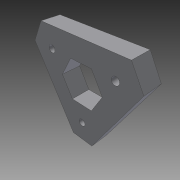
# Autodesk Inventor part: spool_hex_holder
Saved by Autodesk Inventor 2014 (Build 180170000, 170)
## iProperties
Created: 2014-04-15
Part Number: spool_hex_holder
Material: Plywood, Finish
Document SubType Name: Modeling
Designer: buben
Density: 0.552 g/cm^3
Appearance: Plywood - New
Author: buben
Autodesk Inventor part; units mm, degrees
ref_plane "YZ Plane" through (0, 0, 0) normal (1, 0, 0) x (0, 1, 0)
ref_plane "XZ Plane" through (0, 0, 0) normal (0, 1, 0) x (-1, 0, 0)
ref_plane "XY Plane" through (0, 0, 0) normal (0, 0, 1) x (1, 0, 0)
sketch "Sketch1" plane through (0, 0, 0) normal (0, 1, 0) x (-1, 0, 0)
  line L0 (-3.7528, 6.5) -> (3.7528, 6.5)
  line L1 (3.7528, 6.5) -> (7.5056, 0)
  line L2 (7.5056, 0) -> (3.7528, -6.5)
  line L3 (3.7528, -6.5) -> (-3.7528, -6.5)
  line L4 (-3.7528, -6.5) -> (-7.5056, 0)
  line L5 (-7.5056, 0) -> (-3.7528, 6.5)
  line L6 (-15.0363, 13.3) -> (15.0363, 13.3)
  line L7 (19.0363, 6.3718) -> (4, -19.6718)
  line L8 (-4, -19.6718) -> (-19.0363, 6.3718)
  line L9 (19.0363, 6.3718) -> (15.0363, 13.3)
  line L10 (-15.0363, 13.3) -> (-19.0363, 6.3718)
  line L11 (-4, -19.6718) -> (4, -19.6718)
  line L12 (23.0363, 13.3) -> (0, 0) construction
  line L13 (0, 0) -> (0, -26.6) construction
  line L14 (0, 0) -> (-23.0363, 13.3) construction
  circle A0 centre (11.2583, 6.5) radius 1.25
  circle A1 centre (-11.2583, 6.5) radius 1.25
  circle A2 centre (0, -13) radius 1.25
  dimension "d0" = 8
  dimension "d1" = 8
  dimension "d2" = 8
  dimension "d3" = 8
  dimension "d4" = 8
  dimension "d5" = 8
  dimension "d7" = 13
  dimension "d8" = 6.8
  dimension "d9" = 2.5
  dimension "d10" = 13
  dimension "d11" = 13
  dimension "d12" = 13
  constraints: 30 end point, 9 point on line, 3 centre point, 2 coincident, 2 equal radius, 2 horizontal, 20 other
  measures "d0" distance of L7.start L12.start
  measures "d1" distance of L6.end L12.start
  measures "d2" distance of L6.start L14.end
  measures "d3" distance of L8.end L14.end
  measures "d4" distance of L8.start L13.end
  measures "d5" distance of L7.end L13.end
  measures "d7" distance between parallel lines of L0 L3
  measures "d8" distance between parallel lines of L6 L0
  measures "d9" diameter of A0
  measures "d10" distance of point (0, 0) A0.centre
  measures "d11" distance of A1.centre point (0, 0)
  measures "d12" distance of point (0, 0) A2.centre
extrude "Extrusion1" add sketch "Sketch1" along normal blind 6.5
equation "\"d1\" = d0"
equation "\"d2\" = d0"
equation "\"d3\" = d2"
equation "\"d4\" = d0"
equation "\"d5\" = d4"
equation "\"d11\" = d10"
equation "\"d12\" = d11"
body "Solid1"
